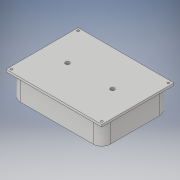
# Autodesk Inventor part: CorollaAirFilterCaseCover
Saved by Autodesk Inventor 2018 (Build 220112000, 112)
## iProperties
Created: 2020-03-28
Part Number: CorollaAirFilterCaseCover
Material: Generic
Document SubType Name: Modeling
Designer: emile
Density: 1 g/cm^3
Appearance: Default
Mass: 925.045 g
Surface Area: 2072.64 cm^2
Volume: 925.045 cm^3
Author: emile
Title: INPUT COVER
Autodesk Inventor part; units mm, degrees
ref_plane "YZ Plane" through (0, 0, 0) normal (1, 0, 0) x (0, 1, 0)
ref_plane "XZ Plane" through (0, 0, 0) normal (0, 1, 0) x (-1, 0, 0)
ref_plane "XY Plane" through (0, 0, 0) normal (0, 0, 1) x (1, 0, 0)
sketch "Sketch1" plane through (0, 0, 0) normal (0, 1, 0) x (-1, 0, 0)
  line L0 (-128.5875, 95.25) -> (128.5875, 95.25)
  line L1 (128.5875, 95.25) -> (128.5875, -95.25)
  line L2 (128.5875, -95.25) -> (-128.5875, -95.25)
  line L3 (-128.5875, -95.25) -> (-128.5875, 95.25)
  line L4 (-128.5875, 95.25) -> (128.5875, -95.25) construction
  line L5 (128.5875, 95.25) -> (-128.5875, -95.25) construction
  line L6 (-115.8875, 82.55) -> (115.8875, 82.55)
  line L7 (115.8875, 82.55) -> (115.8875, -82.55)
  line L8 (115.8875, -82.55) -> (-115.8875, -82.55)
  line L9 (-115.8875, -82.55) -> (-115.8875, 82.55)
  line L10 (-115.8875, 82.55) -> (115.8875, -82.55) construction
  line L11 (115.8875, 82.55) -> (-115.8875, -82.55) construction
  line L12 (134.9375, -101.6) -> (134.9375, 101.6)
  line L13 (134.9375, 101.6) -> (-134.9375, 101.6)
  line L14 (-134.9375, 101.6) -> (-134.9375, -101.6)
  line L15 (-134.9375, -101.6) -> (134.9375, -101.6)
  point P0 (0, 0)
  point P1 (0, 0)
  dimension "d0" = 231.775
  dimension "d1" = 12.7
  dimension "d2" = 12.7
  dimension "d3" = 165.1
  dimension "d4" = 6.35
  constraints: 32 end point, 6 midpoint, 6 parallel, 3 perpendicular, 2 horizontal, 3 other
  measures "d0" distance between parallel lines of L9 L7
  measures "d1" distance between parallel lines of L1 L7
  measures "d2" distance between parallel lines of L2 L8
  measures "d3" distance of L6.end L7.end
  measures "d4" distance between parallel lines of L1 L12
extrude "Extrusion1" add sketch "Sketch1" along normal blind 60 contours L15 L14 L13 L12
extrude "Extrusion2" add sketch "Sketch1" against normal blind 15.24 contours L0 L1 L2 L3 | L6 L7 L8 L9 | L15 L14 L13 L12
fillet "Fillet1" radius 25.4 4 edges at (128.5875, 30, 95.25) (-128.5875, 30, 95.25) (-128.5875, 30, -95.25) (128.5875, 30, -95.25)
sketch "Sketch2" plane through (0, 0, 0) normal (0, 1, 0) x (1, 0, 0)
  line L0 (28.575, -88.9) -> (-28.575, -88.9)
  line L1 (-28.575, 88.9) -> (28.575, 88.9)
  arc A0 (28.575, -88.9) -> (28.575, 88.9) centre (28.575, 0) ccw
  arc A1 (-28.575, 88.9) -> (-28.575, -88.9) centre (-28.575, 0) ccw
  line L2 (28.575, 76.2) -> (-28.575, 76.2)
  arc A2 (-28.575, 76.2) -> (-28.575, -76.2) centre (-28.575, 0) ccw
  line L3 (-28.575, -76.2) -> (28.575, -76.2)
  arc A3 (28.575, -76.2) -> (28.575, 76.2) centre (28.575, 0) ccw
  line L4 (-28.575, 63.5) -> (28.575, 63.5)
  arc A4 (28.575, -63.5) -> (28.575, 63.5) centre (28.575, 0) ccw
  line L5 (28.575, -63.5) -> (-28.575, -63.5)
  arc A5 (-28.575, 63.5) -> (-28.575, -63.5) centre (-28.575, 0) ccw
  line L6 (28.575, 50.8) -> (-28.575, 50.8)
  arc A6 (-28.575, 50.8) -> (-28.575, -50.8) centre (-28.575, 0) ccw
  line L7 (-28.575, -50.8) -> (28.575, -50.8)
  arc A7 (28.575, -50.8) -> (28.575, 50.8) centre (28.575, 0) ccw
  line L8 (-28.575, 38.1) -> (28.575, 38.1)
  arc A8 (28.575, -38.1) -> (28.575, 38.1) centre (28.575, 0) ccw
  line L9 (28.575, -38.1) -> (-28.575, -38.1)
  arc A9 (-28.575, 38.1) -> (-28.575, -38.1) centre (-28.575, 0) ccw
  line L10 (28.575, 25.4) -> (-28.575, 25.4)
  arc A10 (-28.575, 25.4) -> (-28.575, -25.4) centre (-28.575, 0) ccw
  line L11 (-28.575, -25.4) -> (28.575, -25.4)
  arc A11 (28.575, -25.4) -> (28.575, 25.4) centre (28.575, 0) ccw
  line L12 (-28.575, 12.7) -> (28.575, 12.7)
  arc A12 (28.575, -12.7) -> (28.575, 12.7) centre (28.575, 0) ccw
  line L13 (28.575, -12.7) -> (-28.575, -12.7)
  arc A13 (-28.575, 12.7) -> (-28.575, -12.7) centre (-28.575, 0) ccw
  circle A14 centre (0, 0) radius 5.715
  point P0 (0, 12.7)
  dimension "d10" = 88.9
  dimension "d11" = 57.15
  dimension "d12" = 12.7
  dimension "d13" = 12.7
  dimension "d14" = 12.7
  dimension "d15" = 12.7
  dimension "d17" = 12.7
  dimension "d18" = 12.7
  dimension "d19" = 11.43
  constraints: 28 end point, 28 point on circle, 15 centre point, 7 parallel, 4 tangent, 2 horizontal alignment, 1 coincident, 1 midpoint, 1 vertical alignment, 18 other
  measures "d10" radius of A1
  measures "d11" distance of L1.start L1.end
  measures "d12" distance between parallel lines of L1 L2
  measures "d13" distance between parallel lines of L4 L2
  measures "d14" distance between parallel lines of L6 L4
  measures "d15" distance between parallel lines of L8 L10
  measures "d17" distance between parallel lines of L10 L12
  measures "d18" distance between parallel lines of L6 L8
  measures "d19" diameter of A14
extrude "Extrusion3" cut sketch "Sketch2" against normal through all contours A14
extrude "Extrusion4" cut sketch "Sketch2" against normal blind 3.175
sketch "Sketch3" plane through (0, 0, 0) normal (0, 1, 0) x (1, 0, 0)
  arc A0 (128.5875, 69.85) -> (103.1875, 95.25) centre (103.1875, 69.85) ccw projected
  line L0 (103.1875, 95.25) -> (-103.1875, 95.25) projected
  arc A1 (-103.1875, 95.25) -> (-128.5875, 69.85) centre (-103.1875, 69.85) ccw projected
  line L1 (-128.5875, 69.85) -> (-128.5875, -69.85) projected
  arc A2 (-128.5875, -69.85) -> (-103.1875, -95.25) centre (-103.1875, -69.85) ccw projected
  line L2 (-103.1875, -95.25) -> (103.1875, -95.25) projected
  arc A3 (103.1875, -95.25) -> (128.5875, -69.85) centre (103.1875, -69.85) ccw projected
  line L3 (128.5875, -69.85) -> (128.5875, 69.85) projected
  arc A4 (28.575, -88.9) -> (28.575, 88.9) centre (28.575, 0) ccw projected
  line L4 (28.575, -88.9) -> (-28.575, -88.9) projected
  arc A5 (-28.575, 88.9) -> (-28.575, -88.9) centre (-28.575, 0) ccw projected
  line L5 (-28.575, 88.9) -> (28.575, 88.9) projected
  line L6 (-12.7, -88.9) -> (12.7, -88.9)
  line L7 (12.7, -88.9) -> (12.7, 88.9)
  line L8 (12.7, 88.9) -> (-12.7, 88.9)
  line L9 (-12.7, 88.9) -> (-12.7, -88.9)
  line L10 (-12.7, -88.9) -> (12.7, 88.9) construction
  line L11 (12.7, -88.9) -> (-12.7, 88.9) construction
  line L12 (-28.575, 88.9) -> (28.575, 88.9) projected
  line L13 (103.1875, -69.85) -> (-103.1875, 69.85) construction
  circle A6 centre (0, 0) radius 5.715 projected
  line L14 (110.3067, -59.333) -> (-96.0683, 80.367)
  line L15 (-110.3067, 59.333) -> (96.0683, -80.367)
  arc A7 (96.0683, -80.367) -> (110.3067, -59.333) centre (103.1875, -69.85) ccw
  arc A8 (-96.0683, 80.367) -> (-110.3067, 59.333) centre (-103.1875, 69.85) ccw
  line L16 (-103.1875, -69.85) -> (103.1875, 69.85) construction
  line L17 (-96.0683, -80.367) -> (110.3067, 59.333)
  line L18 (96.0683, 80.367) -> (-110.3067, -59.333)
  arc A9 (-110.3067, -59.333) -> (-96.0683, -80.367) centre (-103.1875, -69.85) ccw
  arc A10 (110.3067, 59.333) -> (96.0683, 80.367) centre (103.1875, 69.85) ccw
  dimension "d24" = 25.4
  dimension "d25" = 25.4
  dimension "d26" = 25.4
  constraints: 28 end point, 8 point on circle, 8 tangent, 4 centre point, 4 midpoint, 4 parallel, 2 coincident, 1 horizontal, 1 perpendicular, 1 point on line
  measures "d24" distance between parallel lines of L9 L7
  measures "d25" distance between parallel lines of L18 L17
  measures "d26" distance between parallel lines of L15 L14
extrude "Extrusion5" cut sketch "Sketch3" against normal blind 3.175 contours L15 L7 L17 L14 A4 | A4 L14 A7 L15 | L4 L9 L17 L15 L7 | L15 L17 L7 | L17 L14 L7 L18 A4 | A4 L18 A10 L17 | L17 L7 L14 | L17 L15 L9 L18 L14 L7 | L17 L9 L15 | L17 A5 L18 L15 L9 | L14 L18 L7 | L15 L18 L9 | L17 A9 L18 A5 | L18 L14 L9 L5 L7 | L18 L9 L14 | L18 L15 A5 L14 L9 | L15 A8 L14 A5 | A6
sketch "Sketch4" plane through (0, 0, 0) normal (0, 1, 0) x (1, 0, 0)
  line L0 (-12.7, 23.9331) -> (-12.7, 25.4) projected
  line L1 (-12.7, 25.4) -> (-14.8671, 25.4) projected
  line L2 (-14.8671, 25.4) -> (-12.7, 23.9331) projected
  line L3 (12.7, 23.9331) -> (14.8671, 25.4) projected
  line L4 (14.8671, 25.4) -> (12.7, 25.4) projected
  line L5 (12.7, 25.4) -> (12.7, 23.9331) projected
  line L6 (12.7, -23.9331) -> (12.7, -25.4) projected
  line L7 (12.7, -25.4) -> (14.8671, -25.4) projected
  line L8 (14.8671, -25.4) -> (12.7, -23.9331) projected
  line L9 (-12.7, -25.4) -> (-12.7, -23.9331) projected
  line L10 (-12.7, -23.9331) -> (-14.8671, -25.4) projected
  line L11 (-14.8671, -25.4) -> (-12.7, -25.4) projected
  point P0 (0, 0)
extrude "Extrusion6" cut sketch "Sketch4" against normal blind 3.175
sketch "Sketch5" plane through (0, 60, 0) normal (0, 1, 0) x (1, 0, 0)
  line L0 (-128.5875, -69.85) -> (-128.5875, 69.85) projected
  arc A0 (-103.1875, 95.25) -> (-128.5875, 69.85) centre (-103.1875, 69.85) ccw projected
  line L1 (-103.1875, 95.25) -> (103.1875, 95.25) projected
  arc A1 (128.5875, 69.85) -> (103.1875, 95.25) centre (103.1875, 69.85) ccw projected
  line L2 (128.5875, 69.85) -> (128.5875, -69.85) projected
  arc A2 (103.1875, -95.25) -> (128.5875, -69.85) centre (103.1875, -69.85) ccw projected
  line L3 (103.1875, -95.25) -> (-103.1875, -95.25) projected
  arc A3 (-128.5875, -69.85) -> (-103.1875, -95.25) centre (-103.1875, -69.85) ccw projected
  line L4 (-134.9375, 101.6) -> (-134.9375, -101.6) projected
  line L5 (-134.9375, -101.6) -> (134.9375, -101.6) projected
  line L6 (134.9375, -101.6) -> (134.9375, 101.6) projected
  line L7 (134.9375, 101.6) -> (-134.9375, 101.6) projected
  circle A4 centre (-127.3175, 93.98) radius 3.175
  circle A5 centre (127.3175, 93.98) radius 3.175
  circle A6 centre (127.3175, -93.98) radius 3.175
  circle A7 centre (-127.3175, -93.98) radius 3.175
  point P0 (0, 0)
  dimension "d31" = 6.35
  dimension "d32" = 7.62
  dimension "d33" = 7.62
  dimension "d34" = 7.62
  dimension "d35" = 7.62
  constraints: 4 centre point, 3 equal radius, 2 horizontal alignment, 2 vertical alignment
  measures "d31" diameter of A4
  measures "d32" distance from line of L7 A4.centre
  measures "d33" distance from line of L4 A4.centre
  measures "d34" distance from line of L6 A5.centre
  measures "d35" distance from line of L5 A6.centre
extrude "Extrusion7" cut sketch "Sketch5" against normal through all contours L0 A0 L1 A1 L2 A2 L3 A3 | L7 L6 L5 L4 | A4 | A5 | A6 | A7
extrude "Extrusion8" add sketch "Sketch5" along normal blind 6.35 contours L0 A0 L1 A1 L2 A2 L3 A3 | L7 L6 L5 L4
extrude "Extrusion9" add sketch "Sketch5" against normal blind 6.35 contours L0 A0 L1 A1 L2 A2 L3 A3
sketch "Sketch6" plane through (0, 66.35, 0) normal (0, 1, 0) x (1, 0, 0)
  circle A0 centre (-63.5, 0) radius 5.715
  circle A1 centre (63.5, 0) radius 5.715
  point P0 (0, 0)
  dimension "d42" = 63.5
  dimension "d43" = 63.5
  dimension "d44" = 11.43
  dimension "d45" = 11.43
  constraints: 2 centre point, 2 horizontal alignment
  measures "d42" distance of A0.centre point (0, 0)
  measures "d43" distance of point (0, 0) A1.centre
  measures "d44" diameter of A0
  measures "d45" diameter of A1
extrude "Extrusion10" cut sketch "Sketch6" against normal through all
chamfer "Chamfer2" distance 1.5875 angle 45 8 edges at (0, 53.65, -95.25) (121.148, 53.65, -87.8105) (128.5875, 53.65, 0) (121.148, 53.65, 87.8105) (0, 53.65, 95.25) (-121.148, 53.65, 87.8105) (-128.5875, 53.65, 0) (-121.148, 53.65, -87.8105)
sketch "Sketch7" plane through (0, 53.65, 0) normal (0, -1, 0) x (1, 0, 0)
  circle A0 centre (63.5, 0) radius 5.715 projected
  circle A1 centre (-63.5, 0) radius 5.715 projected
  line L0 (103.1875, -93.6625) -> (-103.1875, -93.6625) projected
  arc A2 (103.1875, -93.6625) -> (127, -69.85) centre (103.1875, -69.85) ccw projected
  line L1 (127, 69.85) -> (127, -69.85) projected
  arc A3 (127, 69.85) -> (103.1875, 93.6625) centre (103.1875, 69.85) ccw projected
  line L2 (-103.1875, 93.6625) -> (103.1875, 93.6625) projected
  arc A4 (-103.1875, 93.6625) -> (-127, 69.85) centre (-103.1875, 69.85) ccw projected
  line L3 (-127, -69.85) -> (-127, 69.85) projected
  arc A5 (-127, -69.85) -> (-103.1875, -93.6625) centre (-103.1875, -69.85) ccw projected
  line L4 (-103.1875, -84.1375) -> (103.1875, -84.1375)
  arc A6 (103.1875, -84.1375) -> (117.475, -69.85) centre (103.1875, -69.85) ccw
  line L5 (117.475, -69.85) -> (117.475, 69.85)
  arc A7 (117.475, 69.85) -> (103.1875, 84.1375) centre (103.1875, 69.85) ccw
  line L6 (103.1875, 84.1375) -> (-103.1875, 84.1375)
  arc A8 (-103.1875, 84.1375) -> (-117.475, 69.85) centre (-103.1875, 69.85) ccw
  line L7 (-117.475, 69.85) -> (-117.475, -69.85)
  arc A9 (-117.475, -69.85) -> (-103.1875, -84.1375) centre (-103.1875, -69.85) ccw
  point P0 (0, 0)
  dimension "d54" = 9.525
  constraints: 8 end point, 8 point on circle, 4 centre point, 7 other
  measures "d54" distance between parallel lines of L0 L4
extrude "Extrusion11" add sketch "Sketch7" along normal blind 55.3466 contours L0 A5 L3 A4 L2 A3 L1 A2
equation "\"d2\" = d1"
equation "\"d13\" = d12"
equation "\"d14\" = d13"
equation "\"d15\" = d14"
equation "\"d17\" = d15"
equation "\"d18\" = d12"
equation "\"d25\" = d24"
equation "\"d26\" = d25"
equation "\"d33\" = d32"
equation "\"d43\" = d42"
equation "\"d45\" = d44"
body "Solid1"
